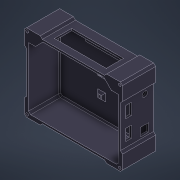
# Autodesk Inventor part: Case
Saved by Autodesk Inventor 2021.1 (Build 251245010, 245A)
## iProperties
Created: 2020-11-26
Part Number: Case
Material: Generic
Document SubType Name: Modeling
Designer: Alex
Density: 1 g/cm^3
Appearance: Default
Author: Alex
Autodesk Inventor part; units mm, degrees
ref_plane "YZ Plane" through (0, 0, 0) normal (1, 0, 0) x (0, 1, 0)
ref_plane "XZ Plane" through (0, 0, 0) normal (0, 1, 0) x (-1, 0, 0)
ref_plane "XY Plane" through (0, 0, 0) normal (0, 0, 1) x (1, 0, 0)
sketch "Sketch1" plane through (0, 0, 0) normal (0, 0, 1) x (1, 0, 0)
  line L0 (-68, 56) -> (-48, 56)
  line L1 (-48, 56) -> (-45, 53)
  line L2 (-45, 53) -> (45, 53)
  line L3 (45, 53) -> (48, 56)
  line L4 (48, 56) -> (68, 56)
  line L5 (68, 56) -> (71, 53)
  line L6 (71, 53) -> (71, 33)
  line L7 (71, 33) -> (68, 30)
  line L8 (68, 30) -> (68, -30)
  line L9 (68, -30) -> (71, -33)
  line L10 (71, -33) -> (71, -53)
  line L11 (71, -53) -> (68, -56)
  line L12 (68, -56) -> (48, -56)
  line L13 (48, -56) -> (45, -53)
  line L14 (45, -53) -> (-45, -53)
  line L15 (-45, -53) -> (-48, -56)
  line L16 (-48, -56) -> (-68, -56)
  line L17 (-68, -56) -> (-71, -53)
  line L18 (-71, -53) -> (-71, -33)
  line L19 (-71, -33) -> (-68, -30)
  line L20 (-68, -30) -> (-68, 30)
  line L21 (-68, 30) -> (-71, 33)
  line L22 (-71, 33) -> (-71, 53)
  line L23 (-71, 53) -> (-68, 56)
  point P0 (0, 0)
  point P1 (-68, 0)
  point P2 (68, 0)
  point P3 (0, -53)
  point P4 (0, 53)
  dimension "d0" = 20
  dimension "d1" = 3
  dimension "d2" = 3
  dimension "d3" = 20
  dimension "d4" = 90
  dimension "d5" = 60
  constraints: 48 end point, 16 parallel, 6 horizontal alignment, 6 vertical alignment, 5 perpendicular, 4 collinear, 4 equal length, 4 midpoint, 2 horizontal, 2 point on line, 2 vertical
  measures "d0" distance of L0.start L0.end
  measures "d1" horizontal distance of L22.end L0.start
  measures "d2" horizontal distance of L22.end L0.start
  measures "d3" distance of L21.end L22.end
  measures "d4" distance of L1.end L2.end
  measures "d5" distance of L19.end L20.end
extrude "Extrusion1" add sketch "Sketch1" along normal blind 3
sketch "Sketch2" plane through (0, 0, 3) normal (0, 0, 1) x (1, 0, 0)
  line L0 (-62, 50) -> (62, 50)
  line L1 (65, 47) -> (65, -47)
  line L2 (62, -50) -> (-62, -50)
  line L3 (-65, -47) -> (-65, 47)
  line L4 (-71, 53) -> (-71, 33) projected
  line L5 (-71, 33) -> (-68, 30) projected
  line L6 (-68, 30) -> (-68, -30) projected
  line L7 (-68, -30) -> (-71, -33) projected
  line L8 (-71, -33) -> (-71, -53) projected
  line L9 (-71, -53) -> (-68, -56) projected
  line L10 (-68, -56) -> (-48, -56) projected
  line L11 (-48, -56) -> (-45, -53) projected
  line L12 (-45, -53) -> (45, -53) projected
  line L13 (45, -53) -> (48, -56) projected
  line L14 (48, -56) -> (68, -56) projected
  line L15 (68, -56) -> (71, -53) projected
  line L16 (71, -53) -> (71, -33) projected
  line L17 (71, -33) -> (68, -30) projected
  line L18 (68, -30) -> (68, 30) projected
  line L19 (68, 30) -> (71, 33) projected
  line L20 (71, 33) -> (71, 53) projected
  line L21 (71, 53) -> (68, 56) projected
  line L22 (68, 56) -> (48, 56) projected
  line L23 (48, 56) -> (45, 53) projected
  line L24 (45, 53) -> (-45, 53) projected
  line L25 (-45, 53) -> (-48, 56) projected
  line L26 (-48, 56) -> (-68, 56) projected
  line L27 (-68, 56) -> (-71, 53) projected
  line L28 (-65, -47) -> (-62, -50)
  line L29 (62, -50) -> (65, -47)
  line L30 (65, 47) -> (62, 50)
  line L31 (-65, 47) -> (-62, 50)
  point P0 (0, 0)
  point P1 (-65, 50)
  point P2 (65, -50)
  point P3 (65, 50)
  point P4 (-65, -50)
  point P5 (0, 50)
  point P6 (-65, 0)
  dimension "d8" = 3
  dimension "d9" = 3
  dimension "d10" = 3
  dimension "d11" = 3
  dimension "d12" = 3
  dimension "d13" = 3
  dimension "d14" = 3
  dimension "d15" = 3
  dimension "d17" = 3
  dimension "d18" = 3
  constraints: 16 end point, 8 point on line, 2 midpoint, 2 parallel, 1 horizontal, 1 horizontal alignment, 1 perpendicular, 1 vertical alignment
  measures "d8" distance between parallel lines of L24 L0
  measures "d9" distance between parallel lines of L6 L3
  measures "d10" distance of L3.start point (-65, -50)
  measures "d11" distance of L2.end point (-65, -50)
  measures "d12" distance of L2.start point (65, -50)
  measures "d13" distance of L1.end point (65, -50)
  measures "d14" distance of L1.start point (65, 50)
  measures "d15" distance of L0.end point (65, 50)
  measures "d17" distance of L0.start point (-65, 50)
  measures "d18" horizontal distance of L3.end L0.start
extrude "Extrusion2" add sketch "Sketch2" along normal blind 45
sketch "Sketch5" plane through (0, 0, 3) normal (0, 0, 1) x (1, 0, 0)
  line L0 (62, -37) -> (-6.6, -37) construction
  line L1 (-6.6, -37) -> (-6.6, 16.3) construction
  line L2 (-6.6, 16.3) -> (62, 16.3) construction
  line L3 (62, 16.3) -> (62, -37) construction
  line L4 (-65, -47) -> (-62, -50) construction
  line L5 (-62, -50) -> (62, -50) construction
  line L6 (62, -50) -> (65, -47) construction
  line L7 (65, -47) -> (65, 47) construction
  line L8 (65, 47) -> (62, 50) construction
  line L9 (62, 50) -> (-62, 50) construction
  line L10 (-62, 50) -> (-65, 47) construction
  line L11 (-65, 47) -> (-65, -47) construction
  line L12 (49.2, -36.9) -> (44.2, -36.9)
  line L13 (44.2, -36.9) -> (44.2, -31.9)
  line L14 (44.2, -31.9) -> (49.2, -31.9)
  line L15 (49.2, -31.9) -> (49.2, -36.9)
  line L16 (49.2, -36.9) -> (44.2, -31.9) construction
  line L17 (44.2, -36.9) -> (49.2, -31.9) construction
  line L18 (-1.6, 6.2) -> (-6.6, 6.2)
  line L19 (-6.6, 6.2) -> (-6.6, 11.2)
  line L20 (-6.6, 11.2) -> (-1.6, 11.2)
  line L21 (-1.6, 11.2) -> (-1.6, 6.2)
  line L22 (-1.6, 6.2) -> (-6.6, 11.2) construction
  line L23 (-6.6, 6.2) -> (-1.6, 11.2) construction
  line L24 (-6.6, -21.7) -> (-1.6, -21.7)
  line L25 (-1.6, -21.7) -> (-1.6, -16.7)
  line L26 (-1.6, -16.7) -> (-6.6, -16.7)
  line L27 (-6.6, -16.7) -> (-6.6, -21.7)
  line L28 (-6.6, -21.7) -> (-1.6, -16.7) construction
  line L29 (-1.6, -21.7) -> (-6.6, -16.7) construction
  line L30 (50.5, 11.3) -> (45.5, 11.3)
  line L31 (45.5, 11.3) -> (45.5, 16.3)
  line L32 (45.5, 16.3) -> (50.5, 16.3)
  line L33 (50.5, 16.3) -> (50.5, 11.3)
  line L34 (50.5, 11.3) -> (45.5, 16.3) construction
  line L35 (45.5, 11.3) -> (50.5, 16.3) construction
  point P0 (0, 0)
  point P1 (46.7, -34.4)
  point P2 (-4.1, -19.2)
  point P3 (48, 13.8)
  point P4 (-4.1, 8.7)
  dimension "d47" = 53.3
  dimension "d48" = 68.6
  dimension "d49" = 13
  dimension "d50" = 3
  dimension "d51" = 14
  dimension "d52" = 1.3
  dimension "d53" = 50.8
  dimension "d54" = 2.5
  dimension "d55" = 5.1
  dimension "d56" = 27.9
  dimension "d57" = 15.2
  dimension "d58" = 5
  dimension "d59" = 5
  constraints: 56 end point, 10 parallel, 8 midpoint, 6 equal length, 5 horizontal, 5 perpendicular, 1 vertical alignment
  measures "d47" distance of L2.end L0.start
  measures "d48" distance of L1.end L2.end
  measures "d49" distance between parallel lines of L5 L0
  measures "d50" distance between parallel lines of L7 L3
  measures "d51" distance from line of L3 point (48, 13.8)
  measures "d52" horizontal distance of point (46.7, -34.4) point (48, 13.8)
  measures "d53" horizontal distance of point (-4.1, -19.2) point (46.7, -34.4)
  measures "d54" distance from line of point (48, 13.8) L2
  measures "d55" vertical distance of point (-4.1, 8.7) point (48, 13.8)
  measures "d56" distance of point (-4.1, -19.2) point (-4.1, 8.7)
  measures "d57" vertical distance of point (46.7, -34.4) point (-4.1, -19.2)
  measures "d58" distance of L13.end L14.end
  measures "d59" distance of L12.end L13.end
extrude "Extrusion6" add sketch "Sketch5" along normal blind 3
chamfer "Chamfer2" distance 3 angle 45 16 edges at (46.7, -31.9, 3) (44.2, -34.4, 3) (46.7, -36.9, 3) (49.2, -34.4, 3) (48, 11.3, 3) (50.5, 13.8, 3) (48, 16.3, 3) (45.5, 13.8, 3) (-4.1, 11.2, 3) (-6.6, 8.7, 3) (-4.1, 6.2, 3) (-1.6, 8.7, 3) (-4.1, -16.7, 3) (-6.6, -19.2, 3) (-4.1, -21.7, 3) (-1.6, -19.2, 3)
sketch "Sketch6" plane through (0, 0, 6) normal (0, 0, 1) x (1, 0, 0)
  point P0 (0, 0)
  point P1 (46.7, -34.4)
  point P2 (48, 13.8)
  point P3 (-4.1, 8.7)
  point P4 (-4.1, -19.2)
hole "Hole1" at (46.7, -34.4, 6) at (48, 13.8, 6) at (-4.1, 8.7, 6) at (-4.1, -19.2, 6) direction (0, 0, -1) diameter 4 depth 5
sketch "Sketch7" plane through (65, -47, 3) normal (-1, 0, 0) x (0, 0, 1)
  line L0 (3, 10) -> (3, 63.3) construction
  line L1 (0, 0) -> (0, 94) construction
  line L2 (0, 0) -> (45, 0) construction
  line L3 (45, 94) -> (45, 0) construction
  line L4 (0, 94) -> (45, 94) construction
  line L5 (3, 63.3) -> (4.6, 63.3) construction
  line L6 (4.6, 63.3) -> (4.6, 0) construction
  line L7 (0, 0) -> (45, 0) construction
  line L8 (15.6, 31.7) -> (4.5, 31.7)
  line L9 (4.5, 31.7) -> (4.5, 19.5)
  line L10 (4.5, 19.5) -> (15.6, 19.5)
  line L11 (15.6, 19.5) -> (15.6, 31.7)
  point P0 (-3, 47)
  point P1 (3, 12.6)
  point P2 (3, 60.8)
  point P3 (0, 10)
  point P4 (0, 63.3)
  dimension "d73" = 1.6
  dimension "d75" = 12.2
  dimension "d76" = 11.1
  dimension "d77" = 0.1
  dimension "d80" = 9.5
  constraints: 14 end point, 2 horizontal, 2 horizontal alignment, 2 parallel, 2 perpendicular, 1 point on line, 1 vertical, 3 other
  measures "d73" distance of L0.end L5.end
  measures "d75" distance of L10.end L8.start
  measures "d76" distance of L8.start L8.end
  measures "d77" distance between parallel lines of L6 L9
  measures "d80" distance from line of L10 L0.start
extrude "Extrusion7" cut sketch "Sketch7" against normal up to surface (3 mm away)
sketch "Sketch8" plane through (-45, 53, 0) normal (0, 1, 0) x (1, 0, 0)
  line L0 (82.6, -38.1) -> (7.4, -38.1)
  line L1 (7.4, -38.1) -> (7.4, -12.9)
  line L2 (7.4, -12.9) -> (82.6, -12.9)
  line L3 (82.6, -12.9) -> (82.6, -38.1)
  line L4 (90, -48) -> (0, -48) construction
  line L5 (90, 0) -> (0, 0) projected
  line L6 (82.6, -25.5) -> (7.4, -25.5) construction
  line L7 (90, 0) -> (90, -48) construction
  line L8 (90, -24) -> (-0.5175, -24) construction
  point P0 (45, 0)
  point P1 (45, -38.1)
  point P2 (45, -48)
  dimension "d81" = 75.2
  dimension "d82" = 25.2
  dimension "d84" = 1.5
  constraints: 12 end point, 5 midpoint, 2 parallel, 2 perpendicular, 1 horizontal, 1 vertical alignment
  measures "d81" distance of L0.start L0.end
  measures "d82" distance of L0.end L1.end
  measures "d84" distance between parallel lines of L6 L8
extrude "Extrusion8" cut sketch "Sketch8" against normal up to surface (3 mm away)
sketch "Sketch9" plane through (0, 0, 3) normal (0, 0, 1) x (1, 0, 0)
  line L0 (65, 36.05) -> (-65, 36.05) construction
  line L1 (-65, 36.05) -> (-65, 39.05) construction
  line L2 (-65, 39.05) -> (65, 39.05) construction
  line L3 (65, 39.05) -> (65, 36.05) construction
  line L4 (-9.6, 14.2) -> (-9.6, 3.2) construction
  line L5 (1.4, 14.2) -> (-9.6, 14.2) construction
  line L6 (1.4, 3.2) -> (1.4, 14.2) construction
  line L7 (-9.6, 3.2) -> (1.4, 3.2) construction
  line L8 (41.2, -28.9) -> (41.2, -39.9) construction
  line L9 (52.2, -28.9) -> (41.2, -28.9) construction
  line L10 (52.2, -39.9) -> (52.2, -28.9) construction
  line L11 (41.2, -39.9) -> (52.2, -39.9) construction
  line L12 (-65, -47) -> (-62, -50) construction
  line L13 (-62, -50) -> (62, -50) construction
  line L14 (62, -50) -> (65, -47) construction
  line L15 (65, -47) -> (65, 47) construction
  line L16 (65, 47) -> (62, 50) construction
  line L17 (62, 50) -> (-62, 50) construction
  line L18 (-62, 50) -> (-65, 47) construction
  line L19 (-65, 47) -> (-65, -47) construction
  line L20 (53.5, 8.3) -> (53.5, 19.3) construction
  line L21 (42.5, 8.3) -> (53.5, 8.3) construction
  line L22 (42.5, 19.3) -> (42.5, 8.3) construction
  line L23 (53.5, 19.3) -> (42.5, 19.3) construction
  line L24 (-9.6, -24.7) -> (1.4, -24.7) construction
  line L25 (-9.6, -13.7) -> (-9.6, -24.7) construction
  line L26 (1.4, -13.7) -> (-9.6, -13.7) construction
  line L27 (1.4, -24.7) -> (1.4, -13.7) construction
  line L28 (-71, 53) -> (-71, 33) construction
  line L29 (-68, 56) -> (-71, 53) construction
  line L30 (-48, 56) -> (-68, 56) construction
  line L31 (-45, 53) -> (-48, 56) construction
  line L32 (45, 53) -> (-45, 53) construction
  line L33 (48, 56) -> (45, 53) construction
  line L34 (68, 56) -> (48, 56) construction
  line L35 (71, 53) -> (68, 56) construction
  line L36 (71, 33) -> (71, 53) construction
  line L37 (68, 30) -> (71, 33) construction
  line L38 (68, -30) -> (68, 30) construction
  line L39 (71, -33) -> (68, -30) construction
  line L40 (71, -53) -> (71, -33) construction
  line L41 (68, -56) -> (71, -53) construction
  line L42 (48, -56) -> (68, -56) construction
  line L43 (45, -53) -> (48, -56) construction
  line L44 (-45, -53) -> (45, -53) construction
  line L45 (-48, -56) -> (-45, -53) construction
  line L46 (-68, -56) -> (-48, -56) construction
  line L47 (-71, -53) -> (-68, -56) construction
  line L48 (-71, -33) -> (-71, -53) construction
  line L49 (-68, -30) -> (-71, -33) construction
  line L50 (-68, 30) -> (-68, -30) construction
  line L51 (-71, 33) -> (-68, 30) construction
  line L52 (25, 39.05) -> (-25, 39.05)
  line L53 (-25, 39.05) -> (-25, 42.05)
  line L54 (-25, 42.05) -> (25, 42.05)
  line L55 (25, 42.05) -> (25, 39.05)
  point P0 (0, 0)
  point P1 (55, 39.05)
  point P2 (-35, 39.05)
  point P3 (-55, 42.05)
  point P4 (0, 42.05)
  dimension "d87" = 3
  dimension "d88" = 13.95
  dimension "d89" = 50
  dimension "d98" = 3
  constraints: 16 end point, 4 parallel, 4 point on line, 2 collinear, 2 horizontal, 2 perpendicular, 1 midpoint, 1 vertical alignment
  measures "d87" distance between parallel lines of L0 L2
  measures "d88" distance between parallel lines of L2 L32
  measures "d89" distance of L53.end L54.end
  measures "d98" distance of L52.end L53.end
extrude "Extrusion9" add sketch "Sketch9" along normal blind 2
chamfer "Chamfer4" distance 2 angle 45 3 edges at (-25, 40.55, 3) (0, 42.05, 3) (25, 40.55, 3)
sketch "Sketch10" plane through (0, 0, 3) normal (0, 0, 1) x (1, 0, 0)
  line L0 (27, 39.05) -> (-27, 39.05) construction
  line L1 (-27, 44.05) -> (-27, 39.05) construction
  line L2 (27, 44.05) -> (-27, 44.05) construction
  line L3 (27, 39.05) -> (27, 44.05) construction
  line L4 (-9.6, 14.2) -> (-9.6, 3.2) construction
  line L5 (1.4, 14.2) -> (-9.6, 14.2) construction
  line L6 (1.4, 3.2) -> (1.4, 14.2) construction
  line L7 (-9.6, 3.2) -> (1.4, 3.2) construction
  line L8 (41.2, -28.9) -> (41.2, -39.9) construction
  line L9 (52.2, -28.9) -> (41.2, -28.9) construction
  line L10 (52.2, -39.9) -> (52.2, -28.9) construction
  line L11 (41.2, -39.9) -> (52.2, -39.9) construction
  line L12 (-65, -47) -> (-62, -50) construction
  line L13 (-62, -50) -> (62, -50) construction
  line L14 (62, -50) -> (65, -47) construction
  line L15 (65, -47) -> (65, 47) construction
  line L16 (65, 47) -> (62, 50) construction
  line L17 (62, 50) -> (-62, 50) construction
  line L18 (-62, 50) -> (-65, 47) projected
  line L19 (-65, 47) -> (-65, -47) construction
  line L20 (53.5, 8.3) -> (53.5, 19.3) construction
  line L21 (42.5, 8.3) -> (53.5, 8.3) construction
  line L22 (42.5, 19.3) -> (42.5, 8.3) construction
  line L23 (53.5, 19.3) -> (42.5, 19.3) construction
  line L24 (-9.6, -24.7) -> (1.4, -24.7) construction
  line L25 (-9.6, -13.7) -> (-9.6, -24.7) construction
  line L26 (1.4, -13.7) -> (-9.6, -13.7) construction
  line L27 (1.4, -24.7) -> (1.4, -13.7) construction
  line L28 (-65, 39.05) -> (-55, 39.05)
  line L29 (-65, 39.05) -> (-65, 47)
  line L30 (-62, 50) -> (-44.05, 50)
  line L31 (0, 50) -> (0, 0) construction
  line L32 (-55, 39.05) -> (-44.05, 50)
  line L33 (62, 50) -> (65, 47)
  line L34 (65, 39.05) -> (55, 39.05)
  line L35 (65, 39.05) -> (65, 47)
  line L36 (62, 50) -> (44.05, 50)
  line L37 (55, 39.05) -> (44.05, 50)
  dimension "d104" = 10
  dimension "d107" = 135
  constraints: 20 end point, 3 symmetric about line, 2 collinear, 2 point on line, 1 horizontal, 1 midpoint, 1 parallel, 1 vertical
  measures "d104" distance of L28.start L28.end
  measures "d107" angle of L28 L32
extrude "Extrusion10" add sketch "Sketch10" along normal up to surface (45 mm away)
sketch "Sketch11" plane through (-65, 39.05, 3) normal (0, -1, 0) x (1, 0, 0)
  line L0 (10, 45) -> (0, 45) construction
  line L1 (0, 0) -> (0, 45) construction
  line L2 (10, 0) -> (0, 0) construction
  line L3 (10, 0) -> (10, 45) construction
  line L4 (130, 45) -> (120, 45) construction
  line L5 (120, 0) -> (120, 45) construction
  line L6 (130, 0) -> (120, 0) construction
  line L7 (130, 45) -> (130, 0) construction
  point P0 (65, -3)
  point P1 (5, 40)
  point P2 (5, 5)
  point P3 (125, 40)
  point P4 (125, 5)
  dimension "d108" = 5
  dimension "d109" = 5
  dimension "d110" = 5
  dimension "d111" = 5
  constraints: 2 horizontal alignment, 2 vertical alignment
  measures "d108" distance from line of L4 point (125, 40)
  measures "d109" distance from line of L7 point (125, 40)
  measures "d110" distance from line of L2 point (5, 5)
  measures "d111" distance from line of L1 point (5, 5)
hole "Hole2" at (-60, 39.05, 43) at (-60, 39.05, 8) at (60, 39.05, 43) at (60, 39.05, 8) direction (0, 1, 0) diameter 4 depth 5
sketch "Sketch12" plane through (0, 0, 48) normal (0, 0, 1) x (1, 0, 0)
  line L0 (-71, 33) -> (-68, 30) construction
  line L1 (-68, 30) -> (-68, -30) construction
  line L2 (-68, -30) -> (-71, -33) construction
  line L3 (-71, -33) -> (-71, -53) construction
  line L4 (-71, -53) -> (-68, -56) construction
  line L5 (-68, -56) -> (-48, -56) construction
  line L6 (-48, -56) -> (-45, -53) construction
  line L7 (-45, -53) -> (45, -53) construction
  line L8 (45, -53) -> (48, -56) construction
  line L9 (48, -56) -> (68, -56) construction
  line L10 (68, -56) -> (71, -53) construction
  line L11 (71, -53) -> (71, -33) construction
  line L12 (71, -33) -> (68, -30) construction
  line L13 (68, -30) -> (68, 30) construction
  line L14 (68, 30) -> (71, 33) construction
  line L15 (71, 33) -> (71, 53) construction
  line L16 (71, 53) -> (68, 56) construction
  line L17 (68, 56) -> (48, 56) construction
  line L18 (48, 56) -> (45, 53) construction
  line L19 (45, 53) -> (-45, 53) construction
  line L20 (-45, 53) -> (-48, 56) construction
  line L21 (-48, 56) -> (-68, 56) construction
  line L22 (-68, 56) -> (-71, 53) construction
  line L23 (-71, 53) -> (-71, 33) construction
  line L24 (-65, -47) -> (-65, 39.05) construction
  line L25 (-55, 39.05) -> (-65, 39.05) construction
  line L26 (-44.05, 50) -> (-55, 39.05) construction
  line L27 (-44.05, 50) -> (44.05, 50) construction
  line L28 (55, 39.05) -> (44.05, 50) construction
  line L29 (65, 39.05) -> (55, 39.05) construction
  line L30 (65, 39.05) -> (65, -47) construction
  line L31 (65, -47) -> (62, -50) construction
  line L32 (62, -50) -> (-62, -50) construction
  line L33 (-62, -50) -> (-65, -47) construction
  line L34 (-67, -52) -> (67, 52) construction
  line L35 (-67, 52) -> (67, -52) construction
  point P0 (0, 0)
  dimension "d119" = 4
  dimension "d120" = 4
  constraints: 4 end point, 2 horizontal alignment, 2 midpoint, 2 vertical alignment
  measures "d119" distance from line of L5 L34.start
  measures "d120" distance from line of L3 L34.start
hole "Hole3" at (-67, 52, 48) at (-67, -52, 48) at (67, -52, 48) at (67, 52, 48) direction (0, 0, -1) diameter 4 depth 5
sketch "Sketch13" plane through (68, -30, 0) normal (1, 0, 0) x (0, 0, -1)
  line L0 (-39.95, 35.85) -> (-32.05, 35.85)
  line L1 (-32.05, 35.85) -> (-32.05, 52.65)
  line L2 (-32.05, 52.65) -> (-39.95, 52.65)
  line L3 (-39.95, 52.65) -> (-39.95, 35.85)
  line L4 (-43, 32.5) -> (-29, 32.5) construction
  line L5 (-29, 32.5) -> (-29, 56) construction
  line L6 (-29, 56) -> (-43, 56) construction
  line L7 (-43, 56) -> (-43, 32.5) construction
  line L8 (-18.6, 14.7) -> (-7.5, 14.7) construction
  line L9 (-7.5, 14.7) -> (-7.5, 2.5) construction
  line L10 (-7.5, 2.5) -> (-18.6, 2.5) construction
  line L11 (-18.6, 2.5) -> (-18.6, 14.7) construction
  line L12 (0, 0) -> (0, 60) construction
  line L13 (0, 60) -> (-48, 60) construction
  line L14 (-48, 0) -> (-48, 60) construction
  line L15 (0, 0) -> (-48, 0) construction
  circle A0 centre (-12.5, 53) radius 3.75
  line L16 (-43, 4) -> (-29, 4) construction
  line L17 (-29, 4) -> (-29, 27.5) construction
  line L18 (-29, 27.5) -> (-43, 27.5) construction
  line L19 (-43, 27.5) -> (-43, 4) construction
  line L20 (-39.95, 7.35) -> (-32.05, 7.35)
  line L21 (-32.05, 7.35) -> (-32.05, 24.15)
  line L22 (-32.05, 24.15) -> (-39.95, 24.15)
  line L23 (-39.95, 24.15) -> (-39.95, 7.35)
  point P0 (0, 30)
  point P1 (-36, 35.85)
  point P2 (-39.95, 44.25)
  point P3 (-43, 44.25)
  point P4 (-36, 32.5)
  point P5 (-18.6, 8.6)
  point P6 (-43, 15.75)
  point P7 (-39.95, 15.75)
  dimension "d128" = 23.5
  dimension "d129" = 14
  dimension "d130" = 7.9
  dimension "d131" = 16.8
  dimension "d136" = 5
  dimension "d137" = 4
  dimension "d142" = 7.5
  dimension "d143" = 12.5
  dimension "d144" = 7
  dimension "d145" = 4
  constraints: 32 end point, 7 midpoint, 4 collinear, 4 equal length, 4 horizontal, 4 parallel, 2 horizontal alignment, 2 perpendicular, 1 centre point, 1 vertical alignment
  measures "d128" distance of L6.end L4.start
  measures "d129" distance of L4.start L4.end
  measures "d130" distance of L0.start L0.end
  measures "d131" distance of L2.end L0.start
  measures "d136" distance between parallel lines of L7 L14
  measures "d137" distance between parallel lines of L6 L13
  measures "d142" diameter of A0
  measures "d143" distance from line of A0.centre L12
  measures "d144" distance from line of L13 A0.centre
  measures "d145" distance between parallel lines of L15 L16
extrude "Extrusion11" cut sketch "Sketch13" against normal blind 10
chamfer "Chamfer5" distance 2 angle 45 8 edges at (0, 50, 3) (-49.525, 44.525, 3) (-65, -3.975, 3) (0, -50, 3) (-63.5, -48.5, 3) (63.5, -48.5, 3) (65, -3.975, 3) (49.525, 44.525, 3)
equation "\"d2\" = d1"
equation "\"d3\" = d0"
equation "\"d9\" = d8"
equation "\"d11\" = d10"
equation "\"d12\" = d10"
equation "\"d13\" = d12"
equation "\"d14\" = d10"
equation "\"d15\" = d14"
equation "\"d17\" = d8"
equation "\"d18\" = d10"
body "Solid1"
